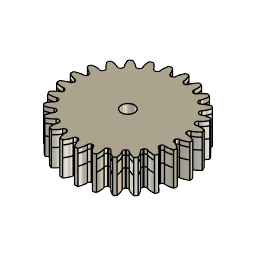
selection_valve_v1 (Autodesk Fusion 360 archive; units mm, degrees)
design "Untitled_Spur Gear 25 teeth"
description: Spur Gear; Module: 2.0; Num Teeth: 25; Pressure Angle: 20.0; Backlash: 0.00 mm
Autodesk Fusion 360 part; units mm, degrees
sketch "Base Circle" plane through (0, 0, 0) normal (0, 0, 1) x (1, 0, 0)
  circle A0 centre (0, 0) radius 22.686
  circle A1 centre (0, 0) radius 3
extrude "Extrude1" add sketch "Base Circle" along normal blind 5
sketch "Gear Tooth" plane through (0, 0, 0) normal (0, 0, 1) x (1, 0, 0)
  spline S0 degree 5 poles (23.4214, -1.8244) (23.4316, -1.8252) (23.4521, -1.8265) (23.4829, -1.8278) (23.524, -1.828) (23.5754, -1.8263) (23.6269, -1.8231) (23.6784, -1.819) (23.7299, -1.8145) (23.7814, -1.8097) (23.833, -1.8045) (23.8845, -1.7988) (23.9361, -1.7926) (23.9876, -1.7857) (24.0392, -1.7781) (24.0907, -1.7699) (24.1423, -1.761) (24.1939, -1.7518) (24.2454, -1.7421) (24.2969, -1.7321) (24.3485, -1.7216) (24.4, -1.7108) (24.4515, -1.6996) (24.503, -1.6879) (24.5544, -1.6758) (24.6059, -1.6633) (24.6573, -1.6504) (24.7087, -1.6371) (24.7602, -1.6235) (24.8115, -1.6095) (24.8629, -1.5952) (24.9142, -1.5805) (24.9655, -1.5655) (25.0168, -1.5501) (25.0681, -1.5344) (25.1193, -1.5184) (25.1706, -1.502) (25.2217, -1.4853) (25.2729, -1.4683) (25.324, -1.451) (25.3751, -1.4333) (25.4262, -1.4154) (25.4772, -1.3971) (25.5282, -1.3786) (25.5792, -1.3597) (25.6301, -1.3406) (25.6811, -1.3211) (25.7319, -1.3014) (25.7828, -1.2814) (25.8336, -1.2611) (25.8843, -1.2405) (25.935, -1.2196) (25.9857, -1.1985) (26.0364, -1.177) (26.087, -1.1553) (26.1375, -1.1334) (26.1881, -1.1111) (26.2386, -1.0886) (26.289, -1.0658) (26.3394, -1.0428) (26.3897, -1.0194) (26.4401, -0.9959) (26.4903, -0.972) (26.5405, -0.948) (26.5907, -0.9236) (26.6409, -0.899) (26.6909, -0.8742) (26.741, -0.849) (26.791, -0.8237) (26.8409, -0.7981) (26.8908, -0.7722) (26.9307, -0.7514) (26.9605, -0.7356) (26.9805, -0.725) (26.9904, -0.7197) knots 0 0 0 0 0 0 0.01428571 0.02857143 0.04285714 0.05714286 0.07142857 0.08571429 0.1 0.11428571 0.12857143 0.14285714 0.15714286 0.17142857 0.18571429 0.2 0.21428571 0.22857143 0.24285714 0.25714286 0.27142857 0.28571429 0.3 0.31428571 0.32857143 0.34285714 0.35714286 0.37142857 0.38571429 0.4 0.41428571 0.42857143 0.44285714 0.45714286 0.47142857 0.48571429 0.5 0.51428571 0.52857143 0.54285714 0.55714286 0.57142857 0.58571429 0.6 0.61428571 0.62857143 0.64285714 0.65714286 0.67142857 0.68571429 0.7 0.71428571 0.72857143 0.74285714 0.75714286 0.77142857 0.78571429 0.8 0.81428571 0.82857143 0.84285714 0.85714286 0.87142857 0.88571429 0.9 0.91428571 0.92857143 0.94285714 0.95714286 0.97142857 0.98571429 1 1 1 1 1 1
  spline S1 degree 5 poles (23.4214, 1.8244) (23.4316, 1.8252) (23.4521, 1.8265) (23.4829, 1.8278) (23.524, 1.828) (23.5754, 1.8263) (23.6269, 1.8231) (23.6784, 1.819) (23.7299, 1.8145) (23.7814, 1.8097) (23.833, 1.8045) (23.8845, 1.7988) (23.9361, 1.7926) (23.9876, 1.7857) (24.0392, 1.7781) (24.0907, 1.7699) (24.1423, 1.761) (24.1939, 1.7518) (24.2454, 1.7421) (24.2969, 1.7321) (24.3485, 1.7216) (24.4, 1.7108) (24.4515, 1.6996) (24.503, 1.6879) (24.5544, 1.6758) (24.6059, 1.6633) (24.6573, 1.6504) (24.7087, 1.6371) (24.7602, 1.6235) (24.8115, 1.6095) (24.8629, 1.5952) (24.9142, 1.5805) (24.9655, 1.5655) (25.0168, 1.5501) (25.0681, 1.5344) (25.1193, 1.5184) (25.1706, 1.502) (25.2217, 1.4853) (25.2729, 1.4683) (25.324, 1.451) (25.3751, 1.4333) (25.4262, 1.4154) (25.4772, 1.3971) (25.5282, 1.3786) (25.5792, 1.3597) (25.6301, 1.3406) (25.6811, 1.3211) (25.7319, 1.3014) (25.7828, 1.2814) (25.8336, 1.2611) (25.8843, 1.2405) (25.935, 1.2196) (25.9857, 1.1985) (26.0364, 1.177) (26.087, 1.1553) (26.1375, 1.1334) (26.1881, 1.1111) (26.2386, 1.0886) (26.289, 1.0658) (26.3394, 1.0428) (26.3897, 1.0194) (26.4401, 0.9959) (26.4903, 0.972) (26.5405, 0.948) (26.5907, 0.9236) (26.6409, 0.899) (26.6909, 0.8742) (26.741, 0.849) (26.791, 0.8237) (26.8409, 0.7981) (26.8908, 0.7722) (26.9307, 0.7514) (26.9605, 0.7356) (26.9805, 0.725) (26.9904, 0.7197) knots 0 0 0 0 0 0 0.01428571 0.02857143 0.04285714 0.05714286 0.07142857 0.08571429 0.1 0.11428571 0.12857143 0.14285714 0.15714286 0.17142857 0.18571429 0.2 0.21428571 0.22857143 0.24285714 0.25714286 0.27142857 0.28571429 0.3 0.31428571 0.32857143 0.34285714 0.35714286 0.37142857 0.38571429 0.4 0.41428571 0.42857143 0.44285714 0.45714286 0.47142857 0.48571429 0.5 0.51428571 0.52857143 0.54285714 0.55714286 0.57142857 0.58571429 0.6 0.61428571 0.62857143 0.64285714 0.65714286 0.67142857 0.68571429 0.7 0.71428571 0.72857143 0.74285714 0.75714286 0.77142857 0.78571429 0.8 0.81428571 0.82857143 0.84285714 0.85714286 0.87142857 0.88571429 0.9 0.91428571 0.92857143 0.94285714 0.95714286 0.97142857 0.98571429 1 1 1 1 1 1
  arc A0 (26.9904, -0.7197) -> (26.9904, 0.7197) centre (0, 0) ccw
  line L0 (22.6075, -1.761) -> (23.4214, -1.8244)
  line L1 (22.6075, 1.761) -> (23.4214, 1.8244)
  line L2 (22.6075, -1.761) -> (22.6075, 1.761)
  point P0 (23.6731, -1.8194)
  point P1 (23.9263, -1.7937)
  point P2 (24.1804, -1.7541)
  point P3 (24.4352, -1.703)
  point P4 (24.6905, -1.6417)
  point P5 (24.9462, -1.5711)
  point P6 (25.2021, -1.4917)
  point P7 (25.458, -1.404)
  point P8 (25.714, -1.3083)
  point P9 (25.9699, -1.205)
  point P10 (26.2255, -1.0944)
  point P11 (26.4809, -0.9765)
  point P12 (26.7359, -0.8515)
  point P13 (23.6731, 1.8194)
  point P14 (23.9263, 1.7937)
  point P15 (24.1804, 1.7541)
  point P16 (24.4352, 1.703)
  point P17 (24.6905, 1.6417)
  point P18 (24.9462, 1.5711)
  point P19 (25.2021, 1.4917)
  point P20 (25.458, 1.404)
  point P21 (25.714, 1.3083)
  point P22 (25.9699, 1.205)
  point P23 (26.2255, 1.0944)
  point P24 (26.4809, 0.9765)
  point P25 (26.7359, 0.8515)
extrude "Extrude2" add sketch "Gear Tooth" along normal blind 5
fillet "Fillet1" radius 1 2 edges at (22.6175, -1.7617, 2.5) (22.6175, 1.7617, 2.5)
pattern_circular "C-Pattern1" count 25 over 360 about axis through (0, 0, 0) along (0, 0, 1) of "Extrude2", "Fillet1"
sketch "Diametrial Pitch Circle" plane through (0, 0, 0) normal (0, 0, 1) x (1, 0, 0)
  circle A0 centre (0, 0) radius 25 construction
move_body "Move1" bodies 1 to x (1, 0, 0) y (0, 1, 0) z (0, 0, 1) at (0, 0, -0.6087)
move_body "Move2" bodies 1 to x (1, 0, 0) y (0, 1, 0) z (0, 0, 1) at (6.6601, 0.1619, 0)
move_body "Move3" bodies 1 to x (0.982613, -0.185667, 0) y (0.185667, 0.982613, 0) z (0, 0, 1) at (0.1237, 1.2358, 0)
extrude "Extrude3" add 1 faces at (22.4536, -2.8187, -0.6087) along direction (0, 0, -1) blind 8 and the other way blind 7

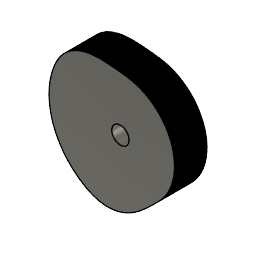
design "cam correct"
Autodesk Fusion 360 part; units mm, degrees
sketch "Sketch1" plane through (0, 0, 0) normal (0, 1, 0) x (1, 0, 0)
  line L0 (63, -36.684) -> (62.9986, -36.4222)
  line L1 (62.9986, -36.4222) -> (62.9945, -36.1605)
  line L2 (62.9945, -36.1605) -> (62.9877, -35.8988)
  line L3 (62.9877, -35.8988) -> (62.9781, -35.6371)
  line L4 (62.9781, -35.6371) -> (62.9657, -35.3756)
  line L5 (62.9657, -35.3756) -> (62.9507, -35.1143)
  line L6 (62.9507, -35.1143) -> (62.9329, -34.8531)
  line L7 (62.9329, -34.8531) -> (62.9123, -34.5921)
  line L8 (62.9123, -34.5921) -> (62.889, -34.3313)
  line L9 (62.889, -34.3313) -> (62.863, -34.0708)
  line L10 (62.863, -34.0708) -> (62.8343, -33.8106)
  line L11 (62.8343, -33.8106) -> (62.8029, -33.5507)
  line L12 (62.8029, -33.5507) -> (62.7687, -33.2912)
  line L13 (62.7687, -33.2912) -> (62.7318, -33.032)
  line L14 (62.7318, -33.032) -> (62.6922, -32.7732)
  line L15 (62.6922, -32.7732) -> (62.6499, -32.5148)
  line L16 (62.6499, -32.5148) -> (62.6049, -32.2569)
  line L17 (62.6049, -32.2569) -> (62.5572, -31.9995)
  line L18 (62.5572, -31.9995) -> (62.5068, -31.7426)
  line L19 (62.5068, -31.7426) -> (62.4537, -31.4862)
  line L20 (62.4537, -31.4862) -> (62.3979, -31.2305)
  line L21 (62.3979, -31.2305) -> (62.3395, -30.9753)
  line L22 (62.3395, -30.9753) -> (62.2784, -30.7207)
  line L23 (62.2784, -30.7207) -> (62.2146, -30.4668)
  line L24 (62.2146, -30.4668) -> (62.1481, -30.2136)
  line L25 (62.1481, -30.2136) -> (62.0791, -29.961)
  line L26 (62.0791, -29.961) -> (62.0073, -29.7093)
  line L27 (62.0073, -29.7093) -> (61.933, -29.4582)
  line L28 (61.933, -29.4582) -> (61.856, -29.208)
  line L29 (61.856, -29.208) -> (61.7764, -28.9586)
  line L30 (61.7764, -28.9586) -> (61.6942, -28.7101)
  line L31 (61.6942, -28.7101) -> (61.6094, -28.4624)
  line L32 (61.6094, -28.4624) -> (61.522, -28.2156)
  line L33 (61.522, -28.2156) -> (61.432, -27.9697)
  line L34 (61.432, -27.9697) -> (61.3395, -27.7248)
  line L35 (61.3395, -27.7248) -> (61.2444, -27.4809)
  line L36 (61.2444, -27.4809) -> (61.1468, -27.238)
  line L37 (61.1468, -27.238) -> (61.0466, -26.9961)
  line L38 (61.0466, -26.9961) -> (60.9439, -26.7553)
  line L39 (60.9439, -26.7553) -> (60.8386, -26.5156)
  line L40 (60.8386, -26.5156) -> (60.7309, -26.277)
  line L41 (60.7309, -26.277) -> (60.6207, -26.0396)
  line L42 (60.6207, -26.0396) -> (60.508, -25.8033)
  line L43 (60.508, -25.8033) -> (60.3928, -25.5682)
  line L44 (60.3928, -25.5682) -> (60.2752, -25.3343)
  line L45 (60.2752, -25.3343) -> (60.1551, -25.1016)
  line L46 (60.1551, -25.1016) -> (60.0326, -24.8703)
  line L47 (60.0326, -24.8703) -> (59.9077, -24.6402)
  line L48 (59.9077, -24.6402) -> (59.7803, -24.4114)
  line L49 (59.7803, -24.4114) -> (59.6506, -24.184)
  line L50 (59.6506, -24.184) -> (59.5186, -23.958)
  line L51 (59.5186, -23.958) -> (59.3841, -23.7334)
  line L52 (59.3841, -23.7334) -> (59.2473, -23.5101)
  line L53 (59.2473, -23.5101) -> (59.1082, -23.2884)
  line L54 (59.1082, -23.2884) -> (58.9668, -23.0681)
  line L55 (58.9668, -23.0681) -> (58.823, -22.8493)
  line L56 (58.823, -22.8493) -> (58.677, -22.632)
  line L57 (58.677, -22.632) -> (58.5287, -22.4162)
  line L58 (58.5287, -22.4162) -> (58.3782, -22.202)
  line L59 (58.3782, -22.202) -> (58.2254, -21.9894)
  line L60 (58.2254, -21.9894) -> (58.0704, -21.7784)
  line L61 (58.0704, -21.7784) -> (57.9132, -21.5691)
  line L62 (57.9132, -21.5691) -> (57.7539, -21.3614)
  line L63 (57.7539, -21.3614) -> (57.5923, -21.1553)
  line L64 (57.5923, -21.1553) -> (57.4286, -20.951)
  line L65 (57.4286, -20.951) -> (57.2628, -20.7484)
  line L66 (57.2628, -20.7484) -> (57.0949, -20.5476)
  line L67 (57.0949, -20.5476) -> (56.9249, -20.3485)
  line L68 (56.9249, -20.3485) -> (56.7531, -20.151)
  line L69 (56.7531, -20.151) -> (56.5795, -19.955)
  line L70 (56.5795, -19.955) -> (56.4044, -19.7604)
  line L71 (56.4044, -19.7604) -> (56.2277, -19.5671)
  line L72 (56.2277, -19.5671) -> (56.0498, -19.3749)
  line L73 (56.0498, -19.3749) -> (55.8706, -19.1839)
  line L74 (55.8706, -19.1839) -> (55.6902, -18.9938)
  line L75 (55.6902, -18.9938) -> (55.5088, -18.8046)
  line L76 (55.5088, -18.8046) -> (55.3264, -18.6162)
  line L77 (55.3264, -18.6162) -> (55.1432, -18.4284)
  line L78 (55.1432, -18.4284) -> (54.959, -18.2412)
  line L79 (54.959, -18.2412) -> (54.7741, -18.0545)
  line L80 (54.7741, -18.0545) -> (54.5884, -17.8682)
  line L81 (54.5884, -17.8682) -> (54.4019, -17.6822)
  line L82 (54.4019, -17.6822) -> (54.2148, -17.4964)
  line L83 (54.2148, -17.4964) -> (54.0269, -17.3108)
  line L84 (54.0269, -17.3108) -> (53.8384, -17.1253)
  line L85 (53.8384, -17.1253) -> (53.6491, -16.9397)
  line L86 (53.6491, -16.9397) -> (53.4592, -16.7541)
  line L87 (53.4592, -16.7541) -> (53.2686, -16.5684)
  line L88 (53.2686, -16.5684) -> (53.0772, -16.3825)
  line L89 (53.0772, -16.3825) -> (52.8851, -16.1964)
  line L90 (52.8851, -16.1964) -> (52.6922, -16.0101)
  line L91 (52.6922, -16.0101) -> (52.4985, -15.8234)
  line L92 (52.4985, -15.8234) -> (52.304, -15.6364)
  line L93 (52.304, -15.6364) -> (52.1085, -15.449)
  line L94 (52.1085, -15.449) -> (51.9121, -15.2612)
  line L95 (51.9121, -15.2612) -> (51.7147, -15.0731)
  line L96 (51.7147, -15.0731) -> (51.5163, -14.8845)
  line L97 (51.5163, -14.8845) -> (51.3167, -14.6955)
  line L98 (51.3167, -14.6955) -> (51.116, -14.5061)
  line L99 (51.116, -14.5061) -> (50.9141, -14.3162)
  line L100 (50.9141, -14.3162) -> (50.7108, -14.126)
  line L101 (50.7108, -14.126) -> (50.5062, -13.9354)
  line L102 (50.5062, -13.9354) -> (50.3001, -13.7444)
  line L103 (50.3001, -13.7444) -> (50.0926, -13.5531)
  line L104 (50.0926, -13.5531) -> (49.8834, -13.3615)
  line L105 (49.8834, -13.3615) -> (49.6727, -13.1696)
  line L106 (49.6727, -13.1696) -> (49.4602, -12.9775)
  line L107 (49.4602, -12.9775) -> (49.2459, -12.7853)
  line L108 (49.2459, -12.7853) -> (49.0297, -12.593)
  line L109 (49.0297, -12.593) -> (48.8117, -12.4006)
  line L110 (48.8117, -12.4006) -> (48.5916, -12.2083)
  line L111 (48.5916, -12.2083) -> (48.3695, -12.0161)
  line L112 (48.3695, -12.0161) -> (48.1452, -11.824)
  line L113 (48.1452, -11.824) -> (47.9187, -11.6323)
  line L114 (47.9187, -11.6323) -> (47.69, -11.4408)
  line L115 (47.69, -11.4408) -> (47.4589, -11.2499)
  line L116 (47.4589, -11.2499) -> (47.2254, -11.0594)
  line L117 (47.2254, -11.0594) -> (46.9895, -10.8696)
  line L118 (46.9895, -10.8696) -> (46.7511, -10.6806)
  line L119 (46.7511, -10.6806) -> (46.5102, -10.4924)
  line L120 (46.5102, -10.4924) -> (46.2666, -10.3052)
  line L121 (46.2666, -10.3052) -> (46.0204, -10.119)
  line L122 (46.0204, -10.119) -> (45.7716, -9.9341)
  line L123 (45.7716, -9.9341) -> (45.52, -9.7505)
  line L124 (45.52, -9.7505) -> (45.2656, -9.5684)
  line L125 (45.2656, -9.5684) -> (45.0085, -9.3878)
  line L126 (45.0085, -9.3878) -> (44.7485, -9.2089)
  line L127 (44.7485, -9.2089) -> (44.4857, -9.0319)
  line L128 (44.4857, -9.0319) -> (44.2201, -8.8569)
  line L129 (44.2201, -8.8569) -> (43.9516, -8.684)
  line L130 (43.9516, -8.684) -> (43.6802, -8.5133)
  line L131 (43.6802, -8.5133) -> (43.406, -8.345)
  line L132 (43.406, -8.345) -> (43.1288, -8.1793)
  line L133 (43.1288, -8.1793) -> (42.8488, -8.0162)
  line L134 (42.8488, -8.0162) -> (42.5659, -7.856)
  line L135 (42.5659, -7.856) -> (42.2802, -7.6987)
  line L136 (42.2802, -7.6987) -> (41.9916, -7.5445)
  line L137 (41.9916, -7.5445) -> (41.7002, -7.3936)
  line L138 (41.7002, -7.3936) -> (41.4061, -7.246)
  line L139 (41.4061, -7.246) -> (41.1092, -7.102)
  line L140 (41.1092, -7.102) -> (40.8096, -6.9616)
  line L141 (40.8096, -6.9616) -> (40.5073, -6.8251)
  line L142 (40.5073, -6.8251) -> (40.2024, -6.6924)
  line L143 (40.2024, -6.6924) -> (39.895, -6.5639)
  line L144 (39.895, -6.5639) -> (39.585, -6.4396)
  line L145 (39.585, -6.4396) -> (39.2726, -6.3196)
  line L146 (39.2726, -6.3196) -> (38.9579, -6.2041)
  line L147 (38.9579, -6.2041) -> (38.6408, -6.0932)
  line L148 (38.6408, -6.0932) -> (38.3215, -5.987)
  line L149 (38.3215, -5.987) -> (38, -5.8857)
  line L150 (38, -5.8857) -> (37.6765, -5.7893)
  line L151 (37.6765, -5.7893) -> (37.3509, -5.698)
  line L152 (37.3509, -5.698) -> (37.0235, -5.6119)
  line L153 (37.0235, -5.6119) -> (36.6943, -5.5311)
  line L154 (36.6943, -5.5311) -> (36.3634, -5.4556)
  line L155 (36.3634, -5.4556) -> (36.0309, -5.3856)
  line L156 (36.0309, -5.3856) -> (35.6969, -5.3212)
  line L157 (35.6969, -5.3212) -> (35.3615, -5.2625)
  line L158 (35.3615, -5.2625) -> (35.0248, -5.2095)
  line L159 (35.0248, -5.2095) -> (34.6869, -5.1623)
  line L160 (34.6869, -5.1623) -> (34.348, -5.121)
  line L161 (34.348, -5.121) -> (34.0082, -5.0857)
  line L162 (34.0082, -5.0857) -> (33.6675, -5.0563)
  line L163 (33.6675, -5.0563) -> (33.3262, -5.033)
  line L164 (33.3262, -5.033) -> (32.9843, -5.0159)
  line L165 (32.9843, -5.0159) -> (32.6419, -5.0048)
  line L166 (32.6419, -5.0048) -> (32.2991, -5)
  line L167 (32.2991, -5) -> (31.9562, -5.0014)
  line L168 (31.9562, -5.0014) -> (31.6132, -5.0089)
  line L169 (31.6132, -5.0089) -> (31.2702, -5.0228)
  line L170 (31.2702, -5.0228) -> (30.9273, -5.0428)
  line L171 (30.9273, -5.0428) -> (30.5848, -5.0691)
  line L172 (30.5848, -5.0691) -> (30.2426, -5.1016)
  line L173 (30.2426, -5.1016) -> (29.901, -5.1404)
  line L174 (29.901, -5.1404) -> (29.5599, -5.1853)
  line L175 (29.5599, -5.1853) -> (29.2197, -5.2365)
  line L176 (29.2197, -5.2365) -> (28.8803, -5.2937)
  line L177 (28.8803, -5.2937) -> (28.5418, -5.357)
  line L178 (28.5418, -5.357) -> (28.2044, -5.4263)
  line L179 (28.2044, -5.4263) -> (27.8682, -5.5016)
  line L180 (27.8682, -5.5016) -> (27.5333, -5.5829)
  line L181 (27.5333, -5.5829) -> (27.1997, -5.6699)
  line L182 (27.1997, -5.6699) -> (26.8676, -5.7627)
  line L183 (26.8676, -5.7627) -> (26.5371, -5.8611)
  line L184 (26.5371, -5.8611) -> (26.2081, -5.9651)
  line L185 (26.2081, -5.9651) -> (25.8808, -6.0745)
  line L186 (25.8808, -6.0745) -> (25.5553, -6.1893)
  line L187 (25.5553, -6.1893) -> (25.2316, -6.3093)
  line L188 (25.2316, -6.3093) -> (24.9098, -6.4344)
  line L189 (24.9098, -6.4344) -> (24.5899, -6.5645)
  line L190 (24.5899, -6.5645) -> (24.272, -6.6994)
  line L191 (24.272, -6.6994) -> (23.956, -6.839)
  line L192 (23.956, -6.839) -> (23.642, -6.9831)
  line L193 (23.642, -6.9831) -> (23.3301, -7.1316)
  line L194 (23.3301, -7.1316) -> (23.0201, -7.2844)
  line L195 (23.0201, -7.2844) -> (22.7122, -7.4412)
  line L196 (22.7122, -7.4412) -> (22.4062, -7.6018)
  line L197 (22.4062, -7.6018) -> (22.1023, -7.7662)
  line L198 (22.1023, -7.7662) -> (21.8002, -7.934)
  line L199 (21.8002, -7.934) -> (21.5, -8.1052)
  line L200 (21.5, -8.1052) -> (21.2016, -8.2796)
  line L201 (21.2016, -8.2796) -> (20.9051, -8.457)
  line L202 (20.9051, -8.457) -> (20.6105, -8.6376)
  line L203 (20.6105, -8.6376) -> (20.3177, -8.8212)
  line L204 (20.3177, -8.8212) -> (20.0269, -9.0079)
  line L205 (20.0269, -9.0079) -> (19.7381, -9.1976)
  line L206 (19.7381, -9.1976) -> (19.4512, -9.3904)
  line L207 (19.4512, -9.3904) -> (19.1665, -9.5861)
  line L208 (19.1665, -9.5861) -> (18.8837, -9.7848)
  line L209 (18.8837, -9.7848) -> (18.6031, -9.9865)
  line L210 (18.6031, -9.9865) -> (18.3246, -10.1911)
  line L211 (18.3246, -10.1911) -> (18.0482, -10.3986)
  line L212 (18.0482, -10.3986) -> (17.7741, -10.6089)
  line L213 (17.7741, -10.6089) -> (17.5021, -10.8222)
  line L214 (17.5021, -10.8222) -> (17.2324, -11.0382)
  line L215 (17.2324, -11.0382) -> (16.965, -11.2571)
  line L216 (16.965, -11.2571) -> (16.6999, -11.4788)
  line L217 (16.6999, -11.4788) -> (16.4371, -11.7032)
  line L218 (16.4371, -11.7032) -> (16.1767, -11.9304)
  line L219 (16.1767, -11.9304) -> (15.9187, -12.1603)
  line L220 (15.9187, -12.1603) -> (15.6631, -12.3928)
  line L221 (15.6631, -12.3928) -> (15.4099, -12.6281)
  line L222 (15.4099, -12.6281) -> (15.1593, -12.866)
  line L223 (15.1593, -12.866) -> (14.9111, -13.1064)
  line L224 (14.9111, -13.1064) -> (14.6655, -13.3495)
  line L225 (14.6655, -13.3495) -> (14.4224, -13.5951)
  line L226 (14.4224, -13.5951) -> (14.1819, -13.8433)
  line L227 (14.1819, -13.8433) -> (13.944, -14.094)
  line L228 (13.944, -14.094) -> (13.7088, -14.3471)
  line L229 (13.7088, -14.3471) -> (13.4762, -14.6027)
  line L230 (13.4762, -14.6027) -> (13.2463, -14.8607)
  line L231 (13.2463, -14.8607) -> (13.0192, -15.1212)
  line L232 (13.0192, -15.1212) -> (12.7947, -15.3839)
  line L233 (12.7947, -15.3839) -> (12.5731, -15.649)
  line L234 (12.5731, -15.649) -> (12.3542, -15.9165)
  line L235 (12.3542, -15.9165) -> (12.1381, -16.1862)
  line L236 (12.1381, -16.1862) -> (11.9249, -16.4581)
  line L237 (11.9249, -16.4581) -> (11.7145, -16.7323)
  line L238 (11.7145, -16.7323) -> (11.507, -17.0086)
  line L239 (11.507, -17.0086) -> (11.3024, -17.2871)
  line L240 (11.3024, -17.2871) -> (11.1008, -17.5678)
  line L241 (11.1008, -17.5678) -> (10.9021, -17.8505)
  line L242 (10.9021, -17.8505) -> (10.7063, -18.1353)
  line L243 (10.7063, -18.1353) -> (10.5136, -18.4221)
  line L244 (10.5136, -18.4221) -> (10.3239, -18.711)
  line L245 (10.3239, -18.711) -> (10.1372, -19.0018)
  line L246 (10.1372, -19.0018) -> (9.9535, -19.2945)
  line L247 (9.9535, -19.2945) -> (9.773, -19.5891)
  line L248 (9.773, -19.5891) -> (9.5955, -19.8857)
  line L249 (9.5955, -19.8857) -> (9.4212, -20.184)
  line L250 (9.4212, -20.184) -> (9.2499, -20.4842)
  line L251 (9.2499, -20.4842) -> (9.0819, -20.7862)
  line L252 (9.0819, -20.7862) -> (8.917, -21.0899)
  line L253 (8.917, -21.0899) -> (8.7553, -21.3953)
  line L254 (8.7553, -21.3953) -> (8.5968, -21.7024)
  line L255 (8.5968, -21.7024) -> (8.4415, -22.0111)
  line L256 (8.4415, -22.0111) -> (8.2895, -22.3214)
  line L257 (8.2895, -22.3214) -> (8.1407, -22.6333)
  line L258 (8.1407, -22.6333) -> (7.9952, -22.9468)
  line L259 (7.9952, -22.9468) -> (7.853, -23.2617)
  line L260 (7.853, -23.2617) -> (7.7141, -23.5782)
  line L261 (7.7141, -23.5782) -> (7.5785, -23.896)
  line L262 (7.5785, -23.896) -> (7.4463, -24.2153)
  line L263 (7.4463, -24.2153) -> (7.3174, -24.5359)
  line L264 (7.3174, -24.5359) -> (7.1918, -24.8579)
  line L265 (7.1918, -24.8579) -> (7.0697, -25.1812)
  line L266 (7.0697, -25.1812) -> (6.9509, -25.5057)
  line L267 (6.9509, -25.5057) -> (6.8356, -25.8314)
  line L268 (6.8356, -25.8314) -> (6.7236, -26.1584)
  line L269 (6.7236, -26.1584) -> (6.6151, -26.4865)
  line L270 (6.6151, -26.4865) -> (6.5101, -26.8157)
  line L271 (6.5101, -26.8157) -> (6.4085, -27.146)
  line L272 (6.4085, -27.146) -> (6.3103, -27.4773)
  line L273 (6.3103, -27.4773) -> (6.2156, -27.8097)
  line L274 (6.2156, -27.8097) -> (6.1244, -28.143)
  line L275 (6.1244, -28.143) -> (6.0368, -28.4773)
  line L276 (6.0368, -28.4773) -> (5.9526, -28.8124)
  line L277 (5.9526, -28.8124) -> (5.8719, -29.1485)
  line L278 (5.8719, -29.1485) -> (5.7947, -29.4853)
  line L279 (5.7947, -29.4853) -> (5.7211, -29.823)
  line L280 (5.7211, -29.823) -> (5.6511, -30.1613)
  line L281 (5.6511, -30.1613) -> (5.5845, -30.5005)
  line L282 (5.5845, -30.5005) -> (5.5215, -30.8402)
  line L283 (5.5215, -30.8402) -> (5.4621, -31.1807)
  line L284 (5.4621, -31.1807) -> (5.4063, -31.5217)
  line L285 (5.4063, -31.5217) -> (5.354, -31.8633)
  line L286 (5.354, -31.8633) -> (5.3053, -32.2054)
  line L287 (5.3053, -32.2054) -> (5.2602, -32.548)
  line L288 (5.2602, -32.548) -> (5.2187, -32.8911)
  line L289 (5.2187, -32.8911) -> (5.1808, -33.2346)
  line L290 (5.1808, -33.2346) -> (5.1465, -33.5785)
  line L291 (5.1465, -33.5785) -> (5.1157, -33.9227)
  line L292 (5.1157, -33.9227) -> (5.0886, -34.2672)
  line L293 (5.0886, -34.2672) -> (5.0651, -34.612)
  line L294 (5.0651, -34.612) -> (5.0452, -34.957)
  line L295 (5.0452, -34.957) -> (5.0289, -35.3021)
  line L296 (5.0289, -35.3021) -> (5.0163, -35.6475)
  line L297 (5.0163, -35.6475) -> (5.0072, -35.9929)
  line L298 (5.0072, -35.9929) -> (5.0018, -36.3385)
  line L299 (5.0018, -36.3385) -> (5, -36.684)
  line L300 (5, -36.684) -> (5.0018, -37.0296)
  line L301 (5.0018, -37.0296) -> (5.0072, -37.3751)
  line L302 (5.0072, -37.3751) -> (5.0163, -37.7206)
  line L303 (5.0163, -37.7206) -> (5.0289, -38.0659)
  line L304 (5.0289, -38.0659) -> (5.0452, -38.4111)
  line L305 (5.0452, -38.4111) -> (5.0651, -38.7561)
  line L306 (5.0651, -38.7561) -> (5.0886, -39.1009)
  line L307 (5.0886, -39.1009) -> (5.1157, -39.4454)
  line L308 (5.1157, -39.4454) -> (5.1465, -39.7896)
  line L309 (5.1465, -39.7896) -> (5.1808, -40.1335)
  line L310 (5.1808, -40.1335) -> (5.2187, -40.477)
  line L311 (5.2187, -40.477) -> (5.2602, -40.82)
  line L312 (5.2602, -40.82) -> (5.3053, -41.1627)
  line L313 (5.3053, -41.1627) -> (5.354, -41.5048)
  line L314 (5.354, -41.5048) -> (5.4063, -41.8464)
  line L315 (5.4063, -41.8464) -> (5.4621, -42.1874)
  line L316 (5.4621, -42.1874) -> (5.5215, -42.5278)
  line L317 (5.5215, -42.5278) -> (5.5845, -42.8676)
  line L318 (5.5845, -42.8676) -> (5.6511, -43.2067)
  line L319 (5.6511, -43.2067) -> (5.7211, -43.5451)
  line L320 (5.7211, -43.5451) -> (5.7947, -43.8828)
  line L321 (5.7947, -43.8828) -> (5.8719, -44.2196)
  line L322 (5.8719, -44.2196) -> (5.9526, -44.5556)
  line L323 (5.9526, -44.5556) -> (6.0368, -44.8908)
  line L324 (6.0368, -44.8908) -> (6.1244, -45.2251)
  line L325 (6.1244, -45.2251) -> (6.2156, -45.5584)
  line L326 (6.2156, -45.5584) -> (6.3103, -45.8907)
  line L327 (6.3103, -45.8907) -> (6.4085, -46.2221)
  line L328 (6.4085, -46.2221) -> (6.5101, -46.5524)
  line L329 (6.5101, -46.5524) -> (6.6151, -46.8816)
  line L330 (6.6151, -46.8816) -> (6.7236, -47.2097)
  line L331 (6.7236, -47.2097) -> (6.8356, -47.5366)
  line L332 (6.8356, -47.5366) -> (6.9509, -47.8624)
  line L333 (6.9509, -47.8624) -> (7.0697, -48.1869)
  line L334 (7.0697, -48.1869) -> (7.1918, -48.5102)
  line L335 (7.1918, -48.5102) -> (7.3174, -48.8321)
  line L336 (7.3174, -48.8321) -> (7.4463, -49.1528)
  line L337 (7.4463, -49.1528) -> (7.5786, -49.472)
  line L338 (7.5786, -49.472) -> (7.7145, -49.7898)
  line L339 (7.7145, -49.7898) -> (7.8541, -50.1059)
  line L340 (7.8541, -50.1059) -> (7.9976, -50.4202)
  line L341 (7.9976, -50.4202) -> (8.1451, -50.7327)
  line L342 (8.1451, -50.7327) -> (8.2967, -51.0432)
  line L343 (8.2967, -51.0432) -> (8.4525, -51.3516)
  line L344 (8.4525, -51.3516) -> (8.6126, -51.6577)
  line L345 (8.6126, -51.6577) -> (8.7771, -51.9614)
  line L346 (8.7771, -51.9614) -> (8.9461, -52.2626)
  line L347 (8.9461, -52.2626) -> (9.1196, -52.5612)
  line L348 (9.1196, -52.5612) -> (9.2977, -52.8569)
  line L349 (9.2977, -52.8569) -> (9.4805, -53.1498)
  line L350 (9.4805, -53.1498) -> (9.6679, -53.4396)
  line L351 (9.6679, -53.4396) -> (9.8599, -53.7263)
  line L352 (9.8599, -53.7263) -> (10.0567, -54.0096)
  line L353 (10.0567, -54.0096) -> (10.2581, -54.2896)
  line L354 (10.2581, -54.2896) -> (10.4643, -54.5659)
  line L355 (10.4643, -54.5659) -> (10.6751, -54.8386)
  line L356 (10.6751, -54.8386) -> (10.8906, -55.1076)
  line L357 (10.8906, -55.1076) -> (11.1107, -55.3726)
  line L358 (11.1107, -55.3726) -> (11.3354, -55.6336)
  line L359 (11.3354, -55.6336) -> (11.5646, -55.8905)
  line L360 (11.5646, -55.8905) -> (11.7983, -56.1431)
  line L361 (11.7983, -56.1431) -> (12.0365, -56.3914)
  line L362 (12.0365, -56.3914) -> (12.279, -56.6353)
  line L363 (12.279, -56.6353) -> (12.5258, -56.8747)
  line L364 (12.5258, -56.8747) -> (12.7768, -57.1094)
  line L365 (12.7768, -57.1094) -> (13.0319, -57.3395)
  line L366 (13.0319, -57.3395) -> (13.291, -57.5647)
  line L367 (13.291, -57.5647) -> (13.5541, -57.7852)
  line L368 (13.5541, -57.7852) -> (13.821, -58.0007)
  line L369 (13.821, -58.0007) -> (14.0916, -58.2112)
  line L370 (14.0916, -58.2112) -> (14.3659, -58.4167)
  line L371 (14.3659, -58.4167) -> (14.6436, -58.6171)
  line L372 (14.6436, -58.6171) -> (14.9248, -58.8124)
  line L373 (14.9248, -58.8124) -> (15.2092, -59.0025)
  line L374 (15.2092, -59.0025) -> (15.4967, -59.1873)
  line L375 (15.4967, -59.1873) -> (15.7872, -59.367)
  line L376 (15.7872, -59.367) -> (16.0807, -59.5413)
  line L377 (16.0807, -59.5413) -> (16.3769, -59.7104)
  line L378 (16.3769, -59.7104) -> (16.6756, -59.8741)
  line L379 (16.6756, -59.8741) -> (16.9769, -60.0325)
  line L380 (16.9769, -60.0325) -> (17.2805, -60.1857)
  line L381 (17.2805, -60.1857) -> (17.5864, -60.3335)
  line L382 (17.5864, -60.3335) -> (17.8943, -60.476)
  line L383 (17.8943, -60.476) -> (18.2041, -60.6132)
  line L384 (18.2041, -60.6132) -> (18.5157, -60.7452)
  line L385 (18.5157, -60.7452) -> (18.829, -60.8719)
  line L386 (18.829, -60.8719) -> (19.1437, -60.9934)
  line L387 (19.1437, -60.9934) -> (19.4599, -61.1097)
  line L388 (19.4599, -61.1097) -> (19.7773, -61.2209)
  line L389 (19.7773, -61.2209) -> (20.0958, -61.3271)
  line L390 (20.0958, -61.3271) -> (20.4152, -61.4282)
  line L391 (20.4152, -61.4282) -> (20.7355, -61.5243)
  line L392 (20.7355, -61.5243) -> (21.0565, -61.6156)
  line L393 (21.0565, -61.6156) -> (21.3781, -61.702)
  line L394 (21.3781, -61.702) -> (21.7002, -61.7836)
  line L395 (21.7002, -61.7836) -> (22.0225, -61.8605)
  line L396 (22.0225, -61.8605) -> (22.3451, -61.9328)
  line L397 (22.3451, -61.9328) -> (22.6677, -62.0006)
  line L398 (22.6677, -62.0006) -> (22.9903, -62.064)
  line L399 (22.9903, -62.064) -> (23.3128, -62.123)
  line L400 (23.3128, -62.123) -> (23.635, -62.1777)
  line L401 (23.635, -62.1777) -> (23.9569, -62.2283)
  line L402 (23.9569, -62.2283) -> (24.2783, -62.2749)
  line L403 (24.2783, -62.2749) -> (24.5992, -62.3175)
  line L404 (24.5992, -62.3175) -> (24.9194, -62.3562)
  line L405 (24.9194, -62.3562) -> (25.2388, -62.3913)
  line L406 (25.2388, -62.3913) -> (25.5575, -62.4227)
  line L407 (25.5575, -62.4227) -> (25.8752, -62.4505)
  line L408 (25.8752, -62.4505) -> (26.192, -62.475)
  line L409 (26.192, -62.475) -> (26.5077, -62.4963)
  line L410 (26.5077, -62.4963) -> (26.8222, -62.5143)
  line L411 (26.8222, -62.5143) -> (27.1356, -62.5293)
  line L412 (27.1356, -62.5293) -> (27.4478, -62.5414)
  line L413 (27.4478, -62.5414) -> (27.7587, -62.5507)
  line L414 (27.7587, -62.5507) -> (28.0682, -62.5573)
  line L415 (28.0682, -62.5573) -> (28.3763, -62.5614)
  line L416 (28.3763, -62.5614) -> (28.683, -62.563)
  line L417 (28.683, -62.563) -> (28.9882, -62.5623)
  line L418 (28.9882, -62.5623) -> (29.292, -62.5594)
  line L419 (29.292, -62.5594) -> (29.5942, -62.5544)
  line L420 (29.5942, -62.5544) -> (29.8949, -62.5474)
  line L421 (29.8949, -62.5474) -> (30.1941, -62.5385)
  line L422 (30.1941, -62.5385) -> (30.4916, -62.528)
  line L423 (30.4916, -62.528) -> (30.7877, -62.5157)
  line L424 (30.7877, -62.5157) -> (31.0821, -62.502)
  line L425 (31.0821, -62.502) -> (31.375, -62.4868)
  line L426 (31.375, -62.4868) -> (31.6663, -62.4703)
  line L427 (31.6663, -62.4703) -> (31.956, -62.4526)
  line L428 (31.956, -62.4526) -> (32.2443, -62.4337)
  line L429 (32.2443, -62.4337) -> (32.531, -62.4139)
  line L430 (32.531, -62.4139) -> (32.8162, -62.393)
  line L431 (32.8162, -62.393) -> (33.0999, -62.3713)
  line L432 (33.0999, -62.3713) -> (33.3822, -62.3488)
  line L433 (33.3822, -62.3488) -> (33.663, -62.3256)
  line L434 (33.663, -62.3256) -> (33.9425, -62.3018)
  line L435 (33.9425, -62.3018) -> (34.2207, -62.2774)
  line L436 (34.2207, -62.2774) -> (34.4976, -62.2524)
  line L437 (34.4976, -62.2524) -> (34.7732, -62.227)
  line L438 (34.7732, -62.227) -> (35.0476, -62.2012)
  line L439 (35.0476, -62.2012) -> (35.3208, -62.175)
  line L440 (35.3208, -62.175) -> (35.5929, -62.1485)
  line L441 (35.5929, -62.1485) -> (35.8639, -62.1216)
  line L442 (35.8639, -62.1216) -> (36.134, -62.0945)
  line L443 (36.134, -62.0945) -> (36.403, -62.0671)
  line L444 (36.403, -62.0671) -> (36.6712, -62.0394)
  line L445 (36.6712, -62.0394) -> (36.9385, -62.0115)
  line L446 (36.9385, -62.0115) -> (37.2049, -61.9833)
  line L447 (37.2049, -61.9833) -> (37.4707, -61.9548)
  line L448 (37.4707, -61.9548) -> (37.7357, -61.926)
  line L449 (37.7357, -61.926) -> (38, -61.8969)
  line L450 (38, -61.8969) -> (38.2637, -61.8675)
  line L451 (38.2637, -61.8675) -> (38.5269, -61.8376)
  line L452 (38.5269, -61.8376) -> (38.7895, -61.8074)
  line L453 (38.7895, -61.8074) -> (39.0517, -61.7766)
  line L454 (39.0517, -61.7766) -> (39.3134, -61.7452)
  line L455 (39.3134, -61.7452) -> (39.5747, -61.7132)
  line L456 (39.5747, -61.7132) -> (39.8356, -61.6805)
  line L457 (39.8356, -61.6805) -> (40.0962, -61.6469)
  line L458 (40.0962, -61.6469) -> (40.3564, -61.6125)
  line L459 (40.3564, -61.6125) -> (40.6164, -61.577)
  line L460 (40.6164, -61.577) -> (40.876, -61.5404)
  line L461 (40.876, -61.5404) -> (41.1353, -61.5025)
  line L462 (41.1353, -61.5025) -> (41.3943, -61.4633)
  line L463 (41.3943, -61.4633) -> (41.6531, -61.4226)
  line L464 (41.6531, -61.4226) -> (41.9115, -61.3802)
  line L465 (41.9115, -61.3802) -> (42.1696, -61.336)
  line L466 (42.1696, -61.336) -> (42.4273, -61.2898)
  line L467 (42.4273, -61.2898) -> (42.6846, -61.2415)
  line L468 (42.6846, -61.2415) -> (42.9414, -61.1909)
  line L469 (42.9414, -61.1909) -> (43.1978, -61.1377)
  line L470 (43.1978, -61.1377) -> (43.4536, -61.082)
  line L471 (43.4536, -61.082) -> (43.7088, -61.0235)
  line L472 (43.7088, -61.0235) -> (43.9633, -60.9624)
  line L473 (43.9633, -60.9624) -> (44.2172, -60.8986)
  line L474 (44.2172, -60.8986) -> (44.4705, -60.8322)
  line L475 (44.4705, -60.8322) -> (44.723, -60.7631)
  line L476 (44.723, -60.7631) -> (44.9748, -60.6914)
  line L477 (44.9748, -60.6914) -> (45.2258, -60.617)
  line L478 (45.2258, -60.617) -> (45.476, -60.54)
  line L479 (45.476, -60.54) -> (45.7254, -60.4605)
  line L480 (45.7254, -60.4605) -> (45.974, -60.3782)
  line L481 (45.974, -60.3782) -> (46.2217, -60.2934)
  line L482 (46.2217, -60.2934) -> (46.4684, -60.2061)
  line L483 (46.4684, -60.2061) -> (46.7143, -60.1161)
  line L484 (46.7143, -60.1161) -> (46.9592, -60.0236)
  line L485 (46.9592, -60.0236) -> (47.2031, -59.9285)
  line L486 (47.2031, -59.9285) -> (47.446, -59.8308)
  line L487 (47.446, -59.8308) -> (47.6879, -59.7306)
  line L488 (47.6879, -59.7306) -> (47.9287, -59.6279)
  line L489 (47.9287, -59.6279) -> (48.1684, -59.5227)
  line L490 (48.1684, -59.5227) -> (48.407, -59.4149)
  line L491 (48.407, -59.4149) -> (48.6445, -59.3047)
  line L492 (48.6445, -59.3047) -> (48.8808, -59.192)
  line L493 (48.8808, -59.192) -> (49.1159, -59.0768)
  line L494 (49.1159, -59.0768) -> (49.3498, -58.9592)
  line L495 (49.3498, -58.9592) -> (49.5824, -58.8391)
  line L496 (49.5824, -58.8391) -> (49.8138, -58.7166)
  line L497 (49.8138, -58.7166) -> (50.0438, -58.5917)
  line L498 (50.0438, -58.5917) -> (50.2726, -58.4644)
  line L499 (50.2726, -58.4644) -> (50.5, -58.3347)
  line L500 (50.5, -58.3347) -> (50.726, -58.2026)
  line L501 (50.726, -58.2026) -> (50.9507, -58.0681)
  line L502 (50.9507, -58.0681) -> (51.1739, -57.9314)
  line L503 (51.1739, -57.9314) -> (51.3957, -57.7922)
  line L504 (51.3957, -57.7922) -> (51.616, -57.6508)
  line L505 (51.616, -57.6508) -> (51.8348, -57.5071)
  line L506 (51.8348, -57.5071) -> (52.0521, -57.3611)
  line L507 (52.0521, -57.3611) -> (52.2678, -57.2128)
  line L508 (52.2678, -57.2128) -> (52.482, -57.0622)
  line L509 (52.482, -57.0622) -> (52.6946, -56.9095)
  line L510 (52.6946, -56.9095) -> (52.9056, -56.7545)
  line L511 (52.9056, -56.7545) -> (53.115, -56.5973)
  line L512 (53.115, -56.5973) -> (53.3227, -56.4379)
  line L513 (53.3227, -56.4379) -> (53.5287, -56.2764)
  line L514 (53.5287, -56.2764) -> (53.733, -56.1127)
  line L515 (53.733, -56.1127) -> (53.9356, -55.9469)
  line L516 (53.9356, -55.9469) -> (54.1364, -55.7789)
  line L517 (54.1364, -55.7789) -> (54.3355, -55.6089)
  line L518 (54.3355, -55.6089) -> (54.5328, -55.4368)
  line L519 (54.5328, -55.4368) -> (54.7283, -55.2627)
  line L520 (54.7283, -55.2627) -> (54.9219, -55.0865)
  line L521 (54.9219, -55.0865) -> (55.1137, -54.9083)
  line L522 (55.1137, -54.9083) -> (55.3036, -54.728)
  line L523 (55.3036, -54.728) -> (55.4916, -54.5459)
  line L524 (55.4916, -54.5459) -> (55.6777, -54.3617)
  line L525 (55.6777, -54.3617) -> (55.8618, -54.1756)
  line L526 (55.8618, -54.1756) -> (56.044, -53.9876)
  line L527 (56.044, -53.9876) -> (56.2242, -53.7977)
  line L528 (56.2242, -53.7977) -> (56.4024, -53.6059)
  line L529 (56.4024, -53.6059) -> (56.5786, -53.4123)
  line L530 (56.5786, -53.4123) -> (56.7528, -53.2168)
  line L531 (56.7528, -53.2168) -> (56.9249, -53.0196)
  line L532 (56.9249, -53.0196) -> (57.0949, -52.8205)
  line L533 (57.0949, -52.8205) -> (57.2628, -52.6196)
  line L534 (57.2628, -52.6196) -> (57.4286, -52.417)
  line L535 (57.4286, -52.417) -> (57.5923, -52.2127)
  line L536 (57.5923, -52.2127) -> (57.7539, -52.0067)
  line L537 (57.7539, -52.0067) -> (57.9132, -51.799)
  line L538 (57.9132, -51.799) -> (58.0704, -51.5897)
  line L539 (58.0704, -51.5897) -> (58.2254, -51.3787)
  line L540 (58.2254, -51.3787) -> (58.3782, -51.1661)
  line L541 (58.3782, -51.1661) -> (58.5287, -50.9519)
  line L542 (58.5287, -50.9519) -> (58.677, -50.7361)
  line L543 (58.677, -50.7361) -> (58.823, -50.5188)
  line L544 (58.823, -50.5188) -> (58.9668, -50.3)
  line L545 (58.9668, -50.3) -> (59.1082, -50.0797)
  line L546 (59.1082, -50.0797) -> (59.2473, -49.8579)
  line L547 (59.2473, -49.8579) -> (59.3841, -49.6347)
  line L548 (59.3841, -49.6347) -> (59.5186, -49.4101)
  line L549 (59.5186, -49.4101) -> (59.6506, -49.184)
  line L550 (59.6506, -49.184) -> (59.7803, -48.9566)
  line L551 (59.7803, -48.9566) -> (59.9077, -48.7279)
  line L552 (59.9077, -48.7279) -> (60.0326, -48.4978)
  line L553 (60.0326, -48.4978) -> (60.1551, -48.2664)
  line L554 (60.1551, -48.2664) -> (60.2752, -48.0338)
  line L555 (60.2752, -48.0338) -> (60.3928, -47.7999)
  line L556 (60.3928, -47.7999) -> (60.508, -47.5648)
  line L557 (60.508, -47.5648) -> (60.6207, -47.3285)
  line L558 (60.6207, -47.3285) -> (60.7309, -47.0911)
  line L559 (60.7309, -47.0911) -> (60.8386, -46.8525)
  line L560 (60.8386, -46.8525) -> (60.9439, -46.6127)
  line L561 (60.9439, -46.6127) -> (61.0466, -46.3719)
  line L562 (61.0466, -46.3719) -> (61.1468, -46.1301)
  line L563 (61.1468, -46.1301) -> (61.2444, -45.8872)
  line L564 (61.2444, -45.8872) -> (61.3395, -45.6432)
  line L565 (61.3395, -45.6432) -> (61.432, -45.3983)
  line L566 (61.432, -45.3983) -> (61.522, -45.1525)
  line L567 (61.522, -45.1525) -> (61.6094, -44.9057)
  line L568 (61.6094, -44.9057) -> (61.6942, -44.658)
  line L569 (61.6942, -44.658) -> (61.7764, -44.4095)
  line L570 (61.7764, -44.4095) -> (61.856, -44.1601)
  line L571 (61.856, -44.1601) -> (61.933, -43.9098)
  line L572 (61.933, -43.9098) -> (62.0073, -43.6588)
  line L573 (62.0073, -43.6588) -> (62.0791, -43.407)
  line L574 (62.0791, -43.407) -> (62.1481, -43.1545)
  line L575 (62.1481, -43.1545) -> (62.2146, -42.9013)
  line L576 (62.2146, -42.9013) -> (62.2784, -42.6474)
  line L577 (62.2784, -42.6474) -> (62.3395, -42.3928)
  line L578 (62.3395, -42.3928) -> (62.3979, -42.1376)
  line L579 (62.3979, -42.1376) -> (62.4537, -41.8818)
  line L580 (62.4537, -41.8818) -> (62.5068, -41.6255)
  line L581 (62.5068, -41.6255) -> (62.5572, -41.3686)
  line L582 (62.5572, -41.3686) -> (62.6049, -41.1112)
  line L583 (62.6049, -41.1112) -> (62.6499, -40.8533)
  line L584 (62.6499, -40.8533) -> (62.6922, -40.5949)
  line L585 (62.6922, -40.5949) -> (62.7318, -40.3361)
  line L586 (62.7318, -40.3361) -> (62.7687, -40.0769)
  line L587 (62.7687, -40.0769) -> (62.8029, -39.8174)
  line L588 (62.8029, -39.8174) -> (62.8343, -39.5575)
  line L589 (62.8343, -39.5575) -> (62.863, -39.2973)
  line L590 (62.863, -39.2973) -> (62.889, -39.0367)
  line L591 (62.889, -39.0367) -> (62.9123, -38.776)
  line L592 (62.9123, -38.776) -> (62.9329, -38.515)
  line L593 (62.9329, -38.515) -> (62.9507, -38.2538)
  line L594 (62.9507, -38.2538) -> (62.9657, -37.9924)
  line L595 (62.9657, -37.9924) -> (62.9781, -37.7309)
  line L596 (62.9781, -37.7309) -> (62.9877, -37.4693)
  line L597 (62.9877, -37.4693) -> (62.9945, -37.2076)
  line L598 (62.9945, -37.2076) -> (62.9986, -36.9458)
  line L599 (62.9986, -36.9458) -> (63, -36.684)
  circle A0 centre (38, -36.684) radius 4
  point P0 (42, -36.684)
extrude "Extrude1" add sketch "Sketch1" along normal blind 15
move_body "Move1" bodies 1 to x (1, 0, 0) y (0, 1, 0) z (0, 0, 1) at (-38, 0, -36.684)
